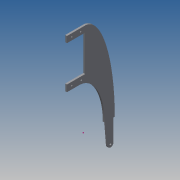
# Autodesk Inventor part: kaki
Saved by Autodesk Inventor 2014 (Build 180170000, 170)
## iProperties
Created: 2015-01-13
Part Number: kaki
Material: Generic
Document SubType Name: Modeling
Designer: I Was ME
Density: 1 g/cm^3
Appearance: Default
Author: I Was ME
Autodesk Inventor part; units mm, degrees
ref_plane "YZ Plane" through (0, 0, 0) normal (1, 0, 0) x (0, 1, 0)
ref_plane "XZ Plane" through (0, 0, 0) normal (0, 1, 0) x (-1, 0, 0)
ref_plane "XY Plane" through (0, 0, 0) normal (0, 0, 1) x (1, 0, 0)
sketch "Sketch1" plane through (0, 0, 0) normal (1, 0, 0) x (0, 1, 0)
  ellipse E0 centre (0, 0) end of major axis (33.5, 0) minor radius 106 (33.5, 0) -> (0, 106) ccw
  line L0 (0, 106) -> (-20.5, 106)
  ellipse E1 centre (-6.5, 0) end of major axis (22, 0) minor radius 51 (22, 0) -> (-6.5, 51) ccw
  line L1 (-20.5, 106) -> (-20.5, 99)
  line L2 (-20.5, 99) -> (0, 99)
  line L3 (0, 99) -> (0, 58.5)
  line L4 (0, 58.5) -> (-20.5, 58.5)
  line L5 (-20.5, 58.5) -> (-20.5, 51)
  line L6 (-20.5, 51) -> (-6.5, 51)
  line L7 (33.5, 0) -> (32, 0)
  line L8 (22, 0) -> (23.5, 0)
  line L9 (0, 106) -> (0, 0) construction
  circle A0 centre (-5, 102.5) radius 0.75
  circle A1 centre (-15, 102.5) radius 0.75
  circle A2 centre (-15, 54.75) radius 0.75
  circle A3 centre (-4.25, 54.75) radius 0.75
  line L10 (23.5, 0) -> (25.5279, -24.9176)
  line L11 (32, 0) -> (32, -24.5)
  circle A4 centre (28.75, -24.4927) radius 3.25
  circle A5 centre (28.75, -24.4927) radius 1
  dimension "d5" = 33.5
  dimension "d6" = 106
  dimension "d12" = 28.5
  dimension "d10" = 20.5
  dimension "d14" = 6.5
  dimension "d15" = 7
  dimension "d16" = 40.5
  dimension "d17" = 1.5
  dimension "d18" = 1.5
  dimension "d22" = 3.5
  dimension "d23" = 5
  dimension "d24" = 1.5
  dimension "d25" = 1.5
  dimension "d26" = 5.5
  dimension "d27" = 1.5
  dimension "d28" = 5.5
  dimension "d29" = 1.5
  dimension "d32" = 25
  dimension "d34" = 24.5
  dimension "d35" = 6.5
  dimension "d36" = 2
  constraints: 24 end point, 6 centre point, 4 parallel, 3 horizontal, 2 coincident, 2 perpendicular, 2 point on circle, 1 collinear, 1 vertical, 8 other
  measures "d10" distance of L0.start L0.end
  measures "d14" distance of point (-6.5, 0) point (0, 0)
  measures "d15" distance of L0.end L1.end
  measures "d16" distance of L2.end L3.end
  measures "d17" distance of L8.start L8.end
  measures "d18" distance of L7.start L7.end
  measures "d22" distance from line of L2 A0.centre
  measures "d23" distance from line of L9 A0.centre
  measures "d24" diameter of A0
  measures "d25" diameter of A1
  measures "d26" distance from line of L1 A1.centre
  measures "d27" diameter of A2
  measures "d28" distance from line of L5 A2.centre
  measures "d29" diameter of A3
  measures "d32" distance of L8.end L10.end
  measures "d34" distance of L7.end L11.end
  measures "d35" diameter of A4
  measures "d36" diameter of A5
sketch "Sketch2" plane through (0, 0, 0) normal (1, 0, 0) x (0, 1, 0)
  point P0 (0, 0)
extrude "Extrusion1" add sketch "Sketch1" along normal blind 2
body "Solid1"
